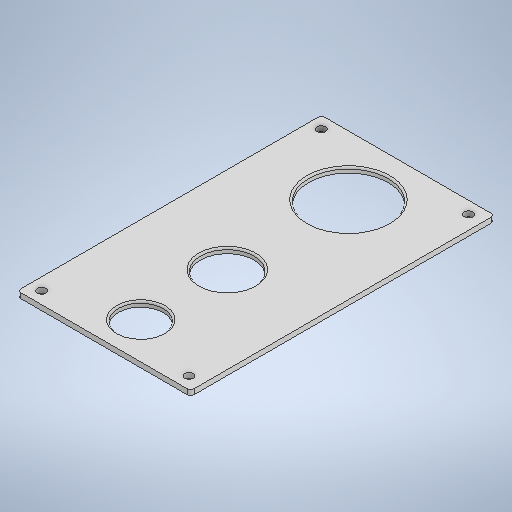
# Autodesk Inventor part: Circle_Color
Saved by Autodesk Inventor 2025 (Build 290162000, 162)
## iProperties
Created: 2026-07-17
Part Number: Circle_Color
Material: Generic
Document SubType Name: Sheet Metal
Designer: MSI
Density: 1 g/cm^3
Sheet Metal Rule: Default_mm
Appearance: Default
Author: MSI
Autodesk Inventor part; units mm, degrees
ref_plane "YZ Plane" through (0, 0, 0) normal (1, 0, 0) x (0, 1, 0)
ref_plane "XZ Plane" through (0, 0, 0) normal (0, 1, 0) x (-1, 0, 0)
ref_plane "XY Plane" through (0, 0, 0) normal (0, 0, 1) x (1, 0, 0)
sketch "Sketch1" plane through (0, 0, 0) normal (0, 1, 0) x (-1, 0, 0)
  circle A0 centre (0, 0) radius 13
  circle A1 centre (0, -50) radius 15.5
  circle A2 centre (0, -120) radius 23
  line L0 (0, 21.1644) -> (-48, 21.1644)
  line L1 (-50, 19.1644) -> (-50, -152.3497)
  line L2 (-48, -154.3497) -> (48, -154.3497)
  line L3 (50, -152.3497) -> (50, 19.1644)
  line L4 (48, 21.1644) -> (0, 21.1644)
  arc A3 (50, 19.1644) -> (48, 21.1644) centre (48, 19.1644) ccw
  arc A4 (-48, 21.1644) -> (-50, 19.1644) centre (-48, 19.1644) ccw
  arc A5 (-50, -152.3497) -> (-48, -154.3497) centre (-48, -152.3497) ccw
  arc A6 (48, -154.3497) -> (50, -152.3497) centre (48, -152.3497) ccw
  point P0 (50, 21.1644)
  constraints: 10 end point, 8 point on circle, 8 tangent, 7 centre point, 3 perpendicular, 3 point on line, 2 equal radius, 1 coincident, 1 collinear, 1 horizontal
extrude "Extrusion1" add sketch "Sketch1" along normal blind 3
fillet "Fillet1" radius 1 3 edges at (13, 3, 0) (15.5, 3, -50) (23, 3, -120)
sketch "Sketch2" plane through (0, 3, 0) normal (0, 1, 0) x (1, 0, 0)
  arc A0 (-50, -19.1644) -> (-48, -21.1644) centre (-48, -19.1644) ccw projected
  circle A1 centre (-43, -14.1644) radius 2.5
  circle A2 centre (-43, 147.3209) radius 2.5
  circle A3 centre (42.0794, -14.1644) radius 2.5
  circle A4 centre (42.0794, 147.3209) radius 2.5
  point P0 (0, 0)
  dimension "d20" = 5
  dimension "d21" = 5
  dimension "d22" = 5
  dimension "d23" = 5
  constraints: 4 centre point
  measures "d20" diameter of A1
  measures "d21" diameter of A2
  measures "d22" diameter of A3
  measures "d23" diameter of A4
extrude "Extrusion2" cut sketch "Sketch2" against normal blind 10
equation "\"BendRadius\" = Thickness"
equation "\"BendReliefWidth\" = Thickness"
equation "\"BendReliefDepth\" = 0.5 * Thickness"
equation "\"CornerReliefSize\" = 4 * Thickness"
equation "\"MinimumRemnant\" = 2 * Thickness"
equation "\"TransitionRadius\" = BendRadius"
equation "\"JacobiRadiusSize\" = BendRadius"
equation "\"GapSize\" = Thickness"
equation "\"Thickness\" = 0.5"
body "Solid1"
